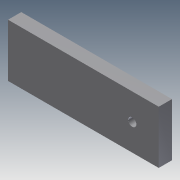
# Autodesk Inventor part: hconnector2
Saved by Autodesk Inventor 2011 (Build 150239000, 239)
## iProperties
Created: 2011-12-11
Part Number: hconnector2
Document SubType Name: Modeling
Designer: Matthew
Density: 1 g/cm^3
Author: Matthew
Autodesk Inventor part; units mm, degrees
ref_plane "YZ Plane" through (0, 0, 0) normal (1, 0, 0) x (0, 1, 0)
ref_plane "XZ Plane" through (0, 0, 0) normal (0, 1, 0) x (-1, 0, 0)
ref_plane "XY Plane" through (0, 0, 0) normal (0, 0, 1) x (1, 0, 0)
sketch "Sketch1" plane through (0, 0, 0) normal (0, 0, 1) x (1, 0, 0)
  line L0 (-53.9057, 15.5084) -> (-1.8807, 15.5084)
  line L1 (-1.8807, 15.5084) -> (-1.8807, -9.8916)
  line L2 (-1.8807, -9.8916) -> (-53.9057, -9.8916)
  line L3 (-53.9057, -9.8916) -> (-53.9057, 15.5084)
  point P0 (0, 0)
  dimension "d0" = 52.025
  dimension "d1" = 25.4
  constraints: 8 end point, 2 parallel, 1 horizontal, 1 perpendicular
  measures "d0" distance of L1.end L2.end
  measures "d1" distance of L0.end L1.end
extrude "Extrusion1" add sketch "Sketch1" along normal blind 6.35
sketch "Sketch2" plane through (-1.8807, -9.8916, 0) normal (1, 0, 0) x (0, 0, -1)
  line L0 (-6.35, 25.4) -> (-6.35, 0) projected
  line L1 (0, 0) -> (-6.35, 0) projected
  line L2 (0, 25.4) -> (0, 0) projected
  line L3 (0, 25.4) -> (-6.35, 25.4) projected
  point P0 (0, 9.8916)
extrude "Extrusion2" add sketch "Sketch2" along normal blind 12.7
sketch "Sketch3" plane through (0, 0, 6.35) normal (0, 0, 1) x (1, 0, 0)
  line L0 (10.8193, -9.8916) -> (10.8193, 15.5084) projected
  line L1 (10.8193, -9.8916) -> (10.8193, 2.8084)
  line L2 (10.8193, 2.8084) -> (-1.8807, 2.8084)
  circle A0 centre (-1.8807, 2.8084) radius 1.9812
  point P0 (0, 0)
  dimension "d6" = 12.7
  dimension "d7" = 3.9624
  constraints: 4 end point, 1 centre point, 1 coincident, 1 midpoint, 1 perpendicular
  measures "d6" distance of L1.end L2.end
  measures "d7" diameter of A0
extrude "Extrusion3" cut sketch "Sketch3" against normal blind 12.7
sketch "Sketch4" plane through (-53.9057, -9.8916, 0) normal (-1, 0, 0) x (0, 0, 1)
  line L0 (6.35, 0) -> (6.35, 25.4) projected
  line L1 (0, 25.4) -> (6.35, 25.4) projected
  line L2 (0, 0) -> (0, 25.4) projected
  line L3 (0, 0) -> (6.35, 0) projected
  point P0 (0, 9.8916)
extrude "Extrusion4" add sketch "Sketch4" along normal blind 6.35
sketch "Sketch5" plane through (-60.2557, -9.8916, 0) normal (-1, 0, 0) x (0, 0, 1)
  line L0 (6.35, 0) -> (0, 0) projected
  line L1 (6.35, 25.4) -> (6.35, 0) projected
  line L2 (0, 25.4) -> (6.35, 25.4) projected
  line L3 (0, 0) -> (0, 25.4) projected
  point P0 (0, 9.8916)
extrude "Extrusion5" add sketch "Sketch5" along normal blind 1.1684
body "Solid1"
